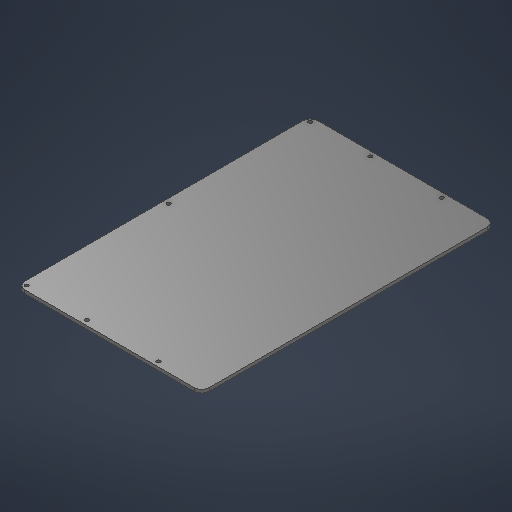
# Autodesk Inventor part: back_plate
Saved by Autodesk Inventor 2026.2 (Build 302298000, 298)
## iProperties
Created: 2026-01-27
Part Number: back_plate
Material: Generic
Document SubType Name: Modeling
Designer: test
Density: 1 g/cm^3
Appearance: Default
Author: test
Autodesk Inventor part; units mm, degrees
ref_plane "YZ Plane" through (0, 0, 0) normal (1, 0, 0) x (0, 1, 0)
ref_plane "XZ Plane" through (0, 0, 0) normal (0, 1, 0) x (-1, 0, 0)
ref_plane "XY Plane" through (0, 0, 0) normal (0, 0, 1) x (1, 0, 0)
sketch "Sketch1" plane through (0, 0, 0) normal (0, 1, 0) x (-1, 0, 0)
  line L0 (0, 0) -> (172.5, 0)
  line L1 (172.5, 0) -> (172.5, -274.11)
  line L2 (172.5, -274.11) -> (0, -274.11)
  line L3 (0, -274.11) -> (0, 0)
  dimension "d0" = 274.11
  dimension "d1" = 172.5
  constraints: 8 end point, 2 parallel, 1 horizontal, 1 perpendicular
  measures "d0" distance between parallel lines of L0 L2
  measures "d1" distance between parallel lines of L3 L1
extrude "Extrusion1" add sketch "Sketch1" along normal blind 3
fillet "Fillet1" radius 7 4 edges at (-172.5, 1.5, 0) (0, 1.5, 0) (-172.5, 1.5, -274.11) (0, 1.5, -274.11)
sketch "Sketch2" plane through (0, 3, 0) normal (0, 1, 0) x (1, 0, 0)
  line L0 (-168, 4.5) -> (-45, 4.5) construction
  line L1 (-45, 4.5) -> (-45, 269.61) construction
  line L2 (-45, 269.61) -> (-168, 269.61) construction
  line L3 (-168, 269.61) -> (-168, 4.5) construction
  line L4 (-172.5, 267.11) -> (-172.5, 7) projected
  line L5 (-172.5, 137.055) -> (0, 137.055) construction
  line L6 (0, 7) -> (0, 267.11) projected
  line L7 (-7, 274.11) -> (-165.5, 274.11) projected
  line L8 (-86.25, 274.11) -> (-86.25, 0) construction
  line L9 (-165.5, 0) -> (-7, 0) projected
  line L10 (-112, 269.61) -> (-112, 4.5) construction
  point P0 (0, 0)
  point P1 (-168, 137.055)
  point P2 (-168, 137.055)
  dimension "d12" = 265.11
  dimension "d13" = 4.5
  dimension "d14" = 123
  dimension "d15" = 67
  constraints: 14 end point, 5 midpoint, 3 coincident, 3 parallel, 3 point on line, 1 horizontal, 1 perpendicular
  measures "d12" distance between parallel lines of L0 L2
  measures "d13" distance between parallel lines of L4 L3
  measures "d14" distance between parallel lines of L3 L1
  measures "d15" distance from line of L1 L10.start
hole "Hole1" at (-168, 3, -4.5) at (-112, 3, -4.5) at (-45, 3, -4.5) at (-168, 3, -137.055) at (-168, 3, -269.61) at (-112, 3, -269.61) at (-45, 3, -269.61) direction (0, -1, 0) diameter 3.5 depth 3
body "Solid1"
